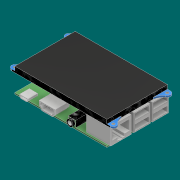
# Autodesk Inventor part: LCD
Saved by Autodesk Inventor 2018 (Build 220112000, 112)
## iProperties
Created: 2019-02-15
Part Number: LCD
Material: Generic
Document SubType Name: Modeling
Designer: Santiago
Density: 1 g/cm^3
Appearance: Default
Author: Santiago
Autodesk Inventor part; units mm, degrees
ref_plane "YZ Plane" through (0, 0, 0) normal (1, 0, 0) x (0, 1, 0)
ref_plane "XZ Plane" through (0, 0, 0) normal (0, 1, 0) x (-1, 0, 0)
sketch "Sketch1" plane through (0, 0, 0) normal (0, 0, 1) x (1, 0, 0)
  line L0 (0, 0) -> (85.5, 0)
  line L1 (85.5, 0) -> (85.5, 56)
  line L2 (85.5, 56) -> (0, 56)
  line L3 (0, 56) -> (0, 0)
  dimension "d0" = 85.5
  dimension "d1" = 56
  dimension "d2" = 85.5
  constraints: 8 end point, 1 horizontal, 1 perpendicular, 1 vertical
  measures "d0" distance of L0.start L0.end
  measures "d1" distance of L0.end L1.end
  measures "d2" distance of L1.end L2.end
extrude "Extrusion1" add sketch "Sketch1" along normal blind 3.7
sketch "Sketch2" plane through (0, 0, 0) normal (0, 0, -1) x (-1, 0, 0)
  line L0 (0, 0) -> (-85.5, 0) projected
  line L1 (-85.5, 0) -> (-85.5, 56) projected
  line L2 (0, 0) -> (-85.5, 0) projected
  line L3 (-42.75, 0) -> (-42.75, -7.3321)
  line L4 (-85.5, 0) -> (-85.5, 56) projected
  line L5 (-85.5, 28) -> (-96.093, 28)
  line L6 (-42.75, 0) -> (-88.35, 0)
  circle A0 centre (-88.35, 3.05) radius 1.25
  circle A1 centre (-88.35, 52.95) radius 1.25
  circle A2 centre (2.85, 3.05) radius 1.25
  circle A3 centre (2.85, 52.95) radius 1.25
  arc A4 (2.85, 0) -> (4.3472, 5.7072) centre (2.85, 3.05) ccw
  line L7 (0, 56) -> (0, 0) projected
  line L8 (0, 56) -> (0, 0) projected
  arc A5 (0, 13.1386) -> (4.3472, 5.7072) centre (13.2145, 15.8817) ccw
  line L9 (2.85, 0) -> (0, 0)
  line L10 (0, 0) -> (0, 13.1386)
  circle A6 centre (-88.35, 3.05) radius 1.25
  arc A7 (-89.8472, 5.7072) -> (-88.35, 0) centre (-88.35, 3.05) ccw
  arc A8 (-89.8472, 5.7072) -> (-85.5, 13.1386) centre (-98.7145, 15.8817) ccw
  line L11 (-88.35, 0) -> (-85.5, 0)
  line L12 (-85.5, 0) -> (-85.5, 13.1386)
  line L13 (-85.5, 56) -> (-85.5, 0)
  line L14 (-42.75, 56) -> (-88.35, 56)
  circle A9 centre (-88.35, 52.95) radius 1.25
  circle A10 centre (2.85, 52.95) radius 1.25
  arc A11 (4.3472, 50.2928) -> (2.85, 56) centre (2.85, 52.95) ccw
  arc A12 (4.3472, 50.2928) -> (0, 42.8614) centre (13.2145, 40.1183) ccw
  line L15 (2.85, 56) -> (0, 56)
  line L16 (0, 56) -> (0, 42.8614)
  line L17 (-88.35, 56) -> (-85.5, 56)
  circle A13 centre (-88.35, 52.95) radius 1.25
  arc A14 (-88.35, 56) -> (-89.8472, 50.2928) centre (-88.35, 52.95) ccw
  arc A15 (-85.5, 42.8614) -> (-89.8472, 50.2928) centre (-98.7145, 40.1183) ccw
  line L18 (-85.5, 42.8614) -> (-85.5, 56)
  line L19 (-88.35, 56) -> (-85.5, 56)
  line L20 (0, 0) -> (-85.5, 0)
  line L21 (-85.5, 0) -> (-85.5, 56)
  line L22 (-85.5, 56) -> (0, 56) projected
  line L23 (-85.5, 56) -> (0, 56)
  line L24 (0, 56) -> (0, 0)
  dimension "d5" = 45.6
  dimension "d7" = 2.5
  constraints: 36 end point, 21 symmetric about line, 16 centre point, 16 point on circle, 5 perpendicular, 4 coincident, 3 collinear, 3 point on line, 2 horizontal, 2 midpoint, 1 tangent, 1 vertical, 13 other
  measures "d5" distance of L3.start L6.end
  measures "d7" diameter of A0
extrude "Extrusion2" add sketch "Sketch2" along normal blind 1.5
ref_plane "Work Plane1" through (0, 0, -17.5) normal (0, 0, -1) x (-1, 0, 0)
sketch "Sketch3" plane through (0, 0, -17.5) normal (0, 0, -1) x (-1, 0, 0)
  line L0 (-88.35, 0) -> (2.85, 0) projected
  line L1 (2.85, 56) -> (-88.35, 56) projected
  line L2 (0, 13.1386) -> (0, 42.8614) projected
  line L3 (-85.5, 42.8614) -> (-85.5, 13.1386) projected
  line L4 (0, 13.1386) -> (0, 0) projected
  line L5 (-85.5, 0) -> (-85.5, 13.1386) projected
  line L6 (-85.5, 42.8614) -> (-85.5, 56) projected
  line L7 (0, 56) -> (0, 42.8614) projected
extrude "Extrusion3" add sketch "Sketch3" along normal blind 1.3
sketch "Sketch4" plane through (0, 0, -17.5) normal (0, 0, 1) x (1, 0, 0)
  line L0 (85.5, 56) -> (0, 56) projected
  line L1 (0, 56) -> (6.8, 56)
  line L2 (6.8, 56) -> (6.8, 55.5)
  line L3 (6.8, 55.5) -> (58.8, 55.5)
  line L4 (58.8, 55.5) -> (58.8, 50.5)
  line L5 (58.8, 50.5) -> (6.8, 50.5)
  line L6 (6.8, 50.5) -> (6.8, 55.5)
  point P0 (0, 0)
  dimension "d13" = 6.8
  dimension "d14" = 0.5
  dimension "d15" = 52
  dimension "d16" = 5
  dimension "d17" = 52
  constraints: 12 end point, 2 perpendicular, 1 horizontal, 1 point on line, 1 vertical
  measures "d13" distance of L0.end L1.end
  measures "d14" distance of L1.end L2.end
  measures "d15" distance of L2.end L3.end
  measures "d16" distance of L3.end L4.end
  measures "d17" distance of L4.end L5.end
extrude "Extrusion4" add sketch "Sketch4" along normal blind 16
sketch "Sketch5" plane through (85.5, 0, -17.5) normal (1, 0, 0) x (0, 0, -1)
  line L0 (0, 0) -> (0, 56) projected
  line L1 (0, 56) -> (0, 55)
  line L2 (0, 55.5) -> (0, 50.5) projected
  line L3 (0, 55) -> (0, 40)
  line L4 (0, 40) -> (-15.9, 40)
  line L5 (-15.9, 40) -> (-15.9, 55)
  line L6 (-15.9, 55) -> (0, 55)
  line L7 (-1, 41) -> (-1, 54)
  line L8 (-14.9, 54) -> (-14.9, 41)
  line L9 (-9.65, 54) -> (-9.65, 41)
  line L10 (-6.25, 54) -> (-6.25, 41)
  line L11 (-14.9, 41) -> (-9.65, 41)
  line L12 (-6.25, 41) -> (-1, 41)
  line L13 (-1, 54) -> (-6.25, 54)
  line L14 (-9.65, 54) -> (-14.9, 54)
  line L15 (0, 40) -> (0, 36.9)
  line L16 (0, 39.0096) -> (0, 38.0096)
  line L17 (0, 38.0096) -> (0, 23.0096)
  line L18 (0, 23.0096) -> (-15.9, 23.0096)
  line L19 (-15.9, 23.0096) -> (-15.9, 38.0096)
  line L20 (-15.9, 38.0096) -> (0, 38.0096)
  line L21 (-1, 24.0096) -> (-1, 37.0096)
  line L22 (-14.9, 37.0096) -> (-14.9, 24.0096)
  line L23 (-9.65, 37.0096) -> (-9.65, 24.0096)
  line L24 (-6.25, 37.0096) -> (-6.25, 24.0096)
  line L25 (-14.9, 24.0096) -> (-9.65, 24.0096)
  line L26 (-6.25, 24.0096) -> (-1, 24.0096)
  line L27 (-1, 37.0096) -> (-6.25, 37.0096)
  line L28 (-9.65, 37.0096) -> (-14.9, 37.0096)
  line L29 (0, 23.0096) -> (0, 19.9096)
  point P0 (-17.5, 0)
  dimension "d20" = 1
  dimension "d21" = 15
  dimension "d22" = 15.9
  dimension "d23" = 15
  dimension "d27" = 3.1
  dimension "d28" = 1
  dimension "d29" = 15
  dimension "d30" = 15.9
  dimension "d31" = 15
  dimension "d32" = 3.1
  constraints: 56 end point, 6 perpendicular, 3 point on line, 2 vertical
  measures "d20" distance of L0.end L1.end
  measures "d21" distance of L1.end L3.end
  measures "d22" distance of L3.end L4.end
  measures "d23" distance of L4.end L5.end
  measures "d27" distance of L3.end L15.end
  measures "d28" distance of L16.start L17.start
  measures "d29" distance of L17.start L17.end
  measures "d30" distance of L17.end L19.start
  measures "d31" distance of L19.start L19.end
  measures "d32" distance of L17.end L29.end
extrude "Extrusion5" add sketch "Sketch5" along normal blind 2
sketch "Sketch6" plane through (87.5, 0, -17.5) normal (1, 0, 0) x (0, 0, -1)
  line L0 (-9.65, 24.0096) -> (-14.9, 24.0096) projected
  line L1 (-14.9, 24.0096) -> (-14.9, 37.0096) projected
  line L2 (-14.9, 37.0096) -> (-9.65, 37.0096) projected
  line L3 (-9.65, 37.0096) -> (-9.65, 24.0096) projected
  line L4 (-1, 24.0096) -> (-6.25, 24.0096) projected
  line L5 (-6.25, 24.0096) -> (-6.25, 37.0096) projected
  line L6 (-6.25, 37.0096) -> (-1, 37.0096) projected
  line L7 (-1, 37.0096) -> (-1, 24.0096) projected
  line L8 (0, 23.0096) -> (0, 38.0096) projected
  line L9 (0, 38.0096) -> (-15.9, 38.0096) projected
  line L10 (-15.9, 38.0096) -> (-15.9, 23.0096) projected
  line L11 (-15.9, 23.0096) -> (0, 23.0096) projected
  line L12 (-1, 41) -> (-6.25, 41) projected
  line L13 (-6.25, 41) -> (-6.25, 54) projected
  line L14 (-6.25, 54) -> (-1, 54) projected
  line L15 (-1, 54) -> (-1, 41) projected
  line L16 (-14.9, 54) -> (-9.65, 54) projected
  line L17 (-9.65, 54) -> (-9.65, 41) projected
  line L18 (-9.65, 41) -> (-14.9, 41) projected
  line L19 (-14.9, 41) -> (-14.9, 54) projected
  line L20 (0, 55) -> (-15.9, 55) projected
  line L21 (-15.9, 55) -> (-15.9, 40) projected
  line L22 (-15.9, 40) -> (0, 40) projected
  line L23 (0, 40) -> (0, 55) projected
  point P0 (-17.5, 0)
extrude "Extrusion6" add sketch "Sketch6" against normal blind 19.1
sketch "Sketch7" plane through (87.5, 0, -17.5) normal (1, 0, 0) x (0, 0, -1)
  line L0 (0, 67.2) -> (0, -11.2) projected
  line L1 (0, 0) -> (0, 23.0096) projected
  line L2 (0, 0) -> (1.3, 0) projected
  line L3 (1.3, 56) -> (1.3, 0) projected
  line L4 (0, 56) -> (1.3, 56) projected
  line L5 (0, 55) -> (0, 56) projected
  line L6 (0, 40) -> (0, 55) projected
  line L7 (0, 38.0096) -> (0, 40) projected
  line L8 (0, 23.0096) -> (0, 38.0096) projected
  line L9 (0, 0) -> (0, 3)
  line L10 (0, 0) -> (0, 23.0096) projected
  line L11 (-3.8, 3) -> (-13.2, 3)
  line L12 (0, 3) -> (0, 19)
  line L13 (-3.8, 19) -> (-13.2, 19)
  line L14 (-15.9, 14.3) -> (-15.9, 3)
  line L15 (-13.2, 19) -> (-13.2, 3)
  line L16 (0, 19) -> (-1.3, 19)
  line L17 (-3.8, 19) -> (-3.8, 14.3)
  line L18 (-3.8, 14.3) -> (-1.3, 14.3)
  line L19 (-1.3, 14.3) -> (-1.3, 12.3)
  line L20 (-1.3, 12.3) -> (-0.65, 12.3)
  line L21 (0, 11) -> (-7.3396, 11)
  line L22 (-3.8, 3) -> (-3.8, 7.7)
  line L23 (-3.8, 7.7) -> (-1.3, 7.7)
  line L24 (-1.3, 7.7) -> (-1.3, 9.7)
  line L25 (-1.3, 9.7) -> (-0.65, 9.7)
  line L26 (0, 3) -> (0, 1.5)
  line L27 (0, 1.5) -> (-15.9, 1.5)
  line L28 (-16, 0) -> (-16, 5.7072) projected
  line L29 (-15.9, 1.5) -> (-15.9, 3)
  line L30 (0, 19) -> (0, 20.5)
  line L31 (0, 20.5) -> (-15.9, 20.5)
  line L32 (-15.9, 20.5) -> (-15.9, 19)
  line L33 (-15.9, 14.3) -> (-15.9, 19)
  line L34 (-16, 42.8614) -> (-16, 13.1386) projected
  line L35 (-13.2, 3) -> (-13.2, 19)
  line L36 (-13.2, 19) -> (-3.8, 19)
  line L37 (-3.8, 14.3) -> (-3.8, 19)
  line L38 (-3.8, 14.3) -> (-1.3, 14.3)
  line L39 (0, 12.3) -> (0, 9.7)
  line L40 (-1.3, 9.7) -> (-0.65, 9.7)
  line L41 (-1.3, 12.3) -> (-0.65, 12.3)
  line L42 (-1.3, 12.3) -> (-1.3, 14.3)
  line L43 (-3.8, 14.3) -> (-1.3, 14.3)
  line L44 (-1.3, 7.7) -> (-1.3, 9.7)
  line L45 (-3.8, 7.7) -> (-1.3, 7.7)
  line L46 (-3.8, 7.7) -> (-3.8, 3)
  line L47 (-13.2, 3) -> (-3.8, 3)
  line L48 (-0.65, 9.7) -> (-0.65, 12.3)
  line L49 (0, 9.7) -> (0, 12.3)
  point P0 (-17.5, 0)
  dimension "d37" = 3
  dimension "d38" = 15.9
  dimension "d39" = 16
  dimension "d40" = 15.9
  dimension "d42" = 3.8
  dimension "d43" = 4.7
  dimension "d44" = 2.5
  dimension "d45" = 2
  dimension "d46" = 1.5
  dimension "d47" = 1.5
  constraints: 76 end point, 15 perpendicular, 10 collinear, 7 point on line, 5 symmetric about line, 1 horizontal, 1 midpoint, 1 parallel
  measures "d37" distance of L1.start L9.end
  measures "d38" distance of L9.end L14.end
  measures "d39" distance of L9.end L12.end
  measures "d40" distance of L12.end L32.end
  measures "d42" distance of L13.start L12.end
  measures "d43" distance of L13.start L17.end
  measures "d44" distance of L17.end L18.end
  measures "d45" distance of L18.end L19.end
  measures "d46" distance of L9.end L26.end
  measures "d47" distance of L12.end L30.end
extrude "Extrusion7" add sketch "Sketch7" against normal blind 21.5 contours L27 L29 L14 L33 L32 L31 L0
sketch "Sketch8" plane through (66, 0, -17.5) normal (-1, 0, 0) x (0, 0, 1)
  line L0 (3.8, 19) -> (13.2, 19) projected
  line L1 (13.2, 19) -> (13.2, 3) projected
  line L2 (13.2, 3) -> (3.8, 3) projected
  line L3 (3.8, 3) -> (3.8, 7.7) projected
  line L4 (3.8, 7.7) -> (1.3, 7.7) projected
  line L5 (1.3, 7.7) -> (1.3, 9.7) projected
  line L6 (1.3, 9.7) -> (0.65, 9.7) projected
  line L7 (0.65, 9.7) -> (0.65, 12.3) projected
  line L8 (0.65, 12.3) -> (1.3, 12.3) projected
  line L9 (1.3, 12.3) -> (1.3, 14.3) projected
  line L10 (1.3, 14.3) -> (3.8, 14.3) projected
  line L11 (3.8, 14.3) -> (3.8, 19) projected
  line L12 (0, 1.5) -> (0, 20.5) projected
  line L13 (0, 1.5) -> (15.9, 1.5) projected
  line L14 (15.9, 1.5) -> (15.9, 20.5) projected
  line L15 (15.9, 20.5) -> (0, 20.5) projected
  point P0 (17.5, 0)
extrude "Extrusion8" add sketch "Sketch8" along normal blind 1 contours L0 L1 L2 L3 L4 L5 L6 L7 L8 L9 L10 L11 | L12 L15 L14 L13
sketch "Sketch9" plane through (68.4, 0, -17.5) normal (-1, 0, 0) x (0, 0, 1)
  line L0 (1, 24.0096) -> (1, 37.0096) projected
  line L1 (1, 37.0096) -> (6.25, 37.0096) projected
  line L2 (6.25, 37.0096) -> (6.25, 24.0096) projected
  line L3 (6.25, 24.0096) -> (1, 24.0096) projected
  line L4 (9.65, 24.0096) -> (9.65, 37.0096) projected
  line L5 (9.65, 37.0096) -> (14.9, 37.0096) projected
  line L6 (14.9, 37.0096) -> (14.9, 24.0096) projected
  line L7 (14.9, 24.0096) -> (9.65, 24.0096) projected
  line L8 (0, 23.0096) -> (0, 38.0096) projected
  line L9 (0, 23.0096) -> (15.9, 23.0096) projected
  line L10 (15.9, 23.0096) -> (15.9, 38.0096) projected
  line L11 (15.9, 38.0096) -> (0, 38.0096) projected
  line L12 (14.9, 54) -> (14.9, 41) projected
  line L13 (14.9, 41) -> (9.65, 41) projected
  line L14 (9.65, 41) -> (9.65, 54) projected
  line L15 (9.65, 54) -> (14.9, 54) projected
  line L16 (1, 41) -> (1, 54) projected
  line L17 (1, 54) -> (6.25, 54) projected
  line L18 (6.25, 54) -> (6.25, 41) projected
  line L19 (6.25, 41) -> (1, 41) projected
  line L20 (15.9, 55) -> (0, 55) projected
  line L21 (0, 40) -> (0, 55) projected
  line L22 (0, 40) -> (15.9, 40) projected
  line L23 (15.9, 40) -> (15.9, 55) projected
  point P0 (17.5, 0)
extrude "Extrusion9" add sketch "Sketch9" along normal blind 1 contours L0 L1 L2 L3 | L4 L5 L6 L7 | L8 L11 L10 L9 | L12 L13 L14 L15 | L16 L17 L18 L19 | L23 L22 L21 L20
sketch "Sketch10" plane through (0, 0, -17.5) normal (0, -1, 0) x (1, 0, 0)
  line L0 (65, 0) -> (65, 15.9) projected
  line L1 (65, 0) -> (56.5, 0)
  line L2 (0, 0) -> (85.5, 0) projected
  line L3 (56.5, 0) -> (56.5, 6)
  line L4 (56.5, 6) -> (49.5, 6)
  line L5 (49.5, 6) -> (49.5, 0)
  line L6 (56.5, 0) -> (49.5, 0)
  line L7 (58.8, 0) -> (6.8, 0) projected
  point P0 (0, 17.5)
  dimension "d54" = 8.5
  dimension "d55" = 6
  dimension "d56" = 7
  constraints: 10 end point, 3 perpendicular, 2 point on line, 1 collinear
  measures "d54" distance of L0.start L1.end
  measures "d55" distance of L1.end L3.end
  measures "d56" distance of L3.end L4.end
extrude "Extrusion10" add sketch "Sketch10" against normal blind 18
sketch "Sketch11" plane through (0, 0, -18.8) normal (0, -1, 0) x (1, 0, 0)
  circle A0 centre (53, 4.3) radius 3
  circle A1 centre (53, 4.3) radius 1.7979
  point P0 (0, 18.8)
  dimension "d59" = 6
  constraints: 2 centre point
  measures "d59" diameter of A0
extrude "Extrusion11" add sketch "Sketch11" along normal blind 2
sketch "Sketch12" plane through (0, 0, -18.8) normal (0, -1, 0) x (1, 0, 0)
  line L0 (49.5, 7.3) -> (49.5, 1.3) projected
  line L1 (49.5, 7.3) -> (49.5, 8.3)
  line L2 (49.5, 8.3) -> (39.5, 8.3)
  line L3 (39.5, 8.3) -> (39.5, 4.3)
  arc A0 (39.5, 4.3) -> (36.9589, 1.3) centre (42.1902, -0.5548) ccw
  line L4 (39.5, 8.3) -> (24.5, 8.3)
  line L5 (24.5, 8.3) -> (24.5, 4.3)
  line L6 (32, 8.3) -> (32, 11.2612)
  arc A1 (27.0411, 1.3) -> (24.5, 4.3) centre (21.8098, -0.5548) ccw
  line L7 (27.0411, 1.3) -> (36.9589, 1.3)
  line L8 (0, 1.3) -> (49.5, 1.3) projected
  line L9 (25.5, 7.3) -> (38.5, 7.3)
  line L10 (38.5, 7.3) -> (38.5, 4.8572)
  arc A2 (38.5, 4.8572) -> (36.2947, 2.3) centre (42.1902, -0.5548) ccw
  line L11 (36.2947, 2.3) -> (27.7053, 2.3)
  arc A3 (27.7053, 2.3) -> (25.5, 4.8572) centre (21.8098, -0.5548) ccw
  line L12 (25.5, 4.8572) -> (25.5, 7.3)
  point P0 (0, 18.8)
  dimension "d62" = 1
  dimension "d63" = 10
  dimension "d64" = 4
  dimension "d65" = 15
  dimension "d66" = 1
  constraints: 22 end point, 8 point on circle, 4 centre point, 4 perpendicular, 2 symmetric about line, 2 vertical, 1 collinear, 1 horizontal, 1 midpoint, 6 other
  measures "d62" distance of L0.start L1.end
  measures "d63" distance of L1.end L2.end
  measures "d64" distance of L2.end L3.end
  measures "d65" distance of L2.end L4.end
  measures "d66" distance between parallel lines of L4 L9
extrude "Extrusion12" add sketch "Sketch12" against normal blind 10 contours L7 A1 L5 L4 L3 A0
sketch "Sketch13" plane through (0, 0, -18.8) normal (0, -1, 0) x (1, 0, 0)
  arc A0 (27.0411, 1.3) -> (24.5, 4.3) centre (21.8098, -0.5548) ccw projected
  line L0 (24.5, 4.3) -> (24.5, 8.3) projected
  line L1 (24.5, 8.3) -> (39.5, 8.3) projected
  line L2 (36.2947, 2.3) -> (27.7053, 2.3) projected
  arc A1 (27.7053, 2.3) -> (25.5, 4.8572) centre (21.8098, -0.5548) ccw projected
  line L3 (25.5, 4.8572) -> (25.5, 7.3) projected
  line L4 (25.5, 7.3) -> (38.5, 7.3) projected
  line L5 (38.5, 7.3) -> (38.5, 4.8572) projected
  arc A2 (38.5, 4.8572) -> (36.2947, 2.3) centre (42.1902, -0.5548) ccw projected
  arc A3 (39.5, 4.3) -> (36.9589, 1.3) centre (42.1902, -0.5548) ccw projected
  line L6 (39.5, 8.3) -> (39.5, 4.3) projected
  arc A4 (27.0411, 1.3) -> (24.5, 4.3) centre (21.8098, -0.5548) ccw projected
  line L7 (36.9589, 1.3) -> (49.5, 1.3) projected
  line L8 (27.0411, 1.3) -> (36.9589, 1.3)
  point P0 (0, 18.8)
  constraints: 2 end point, 1 horizontal
extrude "Extrusion13" add sketch "Sketch13" along normal blind 2
sketch "Sketch14" plane through (0, 10, -18.8) normal (0, 1, 0) x (1, 0, 0)
  line L0 (25.5, -7.3) -> (25.5, -4.8572) projected
  arc A0 (25.5, -4.8572) -> (27.7053, -2.3) centre (21.8098, 0.5548) ccw projected
  line L1 (27.7053, -2.3) -> (36.2947, -2.3) projected
  arc A1 (36.2947, -2.3) -> (38.5, -4.8572) centre (42.1902, 0.5548) ccw projected
  line L2 (38.5, -4.8572) -> (38.5, -7.3) projected
  line L3 (38.5, -7.3) -> (25.5, -7.3) projected
  line L4 (39.5, -8.3) -> (39.5, -4.3) projected
  arc A2 (36.9589, -1.3) -> (39.5, -4.3) centre (42.1902, 0.5548) ccw projected
  line L5 (27.0411, -1.3) -> (36.9589, -1.3) projected
  arc A3 (24.5, -4.3) -> (27.0411, -1.3) centre (21.8098, 0.5548) ccw projected
  line L6 (24.5, -4.3) -> (24.5, -8.3) projected
  line L7 (24.5, -8.3) -> (39.5, -8.3) projected
  point P0 (0, -18.8)
extrude "Extrusion14" add sketch "Sketch14" along normal blind 1 contours L0 A0 L1 A1 L2 L3 | L7 L6 A3 L5 A2 L4
sketch "Sketch15" plane through (0, 10, -18.8) normal (0, -1, 0) x (1, 0, 0)
  line L0 (25.5, 4.8572) -> (25.5, 7.3) projected
  line L1 (38.5, 7.3) -> (38.5, 4.8572) projected
  line L2 (38.5, 4.8572) -> (25.5, 4.8572)
  line L3 (27.7053, 4.8572) -> (27.7053, 5.8572)
  line L4 (27.7053, 5.8572) -> (36.2947, 5.8572)
  line L5 (36.2947, 5.8572) -> (36.2947, 4.8572)
  point P0 (0, 18.8)
  dimension "d73" = 1
  constraints: 8 end point, 2 point on line, 1 horizontal, 1 parallel, 1 perpendicular, 1 vertical
  measures "d73" distance of L3.start L3.end
extrude "Extrusion15" add sketch "Sketch15" along normal blind 10
sketch "Sketch16" plane through (53, 0, -14.5) normal (0, -1, 0) x (1, 0, 0)
  circle A0 centre (0, 0) radius 1.7979 projected
  point P0 (-53, 14.5)
extrude "Extrusion16" cut sketch "Sketch16" against normal blind 10
sketch "Sketch17" plane through (0, -2, -18.8) normal (0, -1, 0) x (1, 0, 0)
  line L0 (24.5, 8.3) -> (24.5, 4.3) projected
  line L1 (24.5, 4.3) -> (14.3, 4.3)
  line L2 (14.3, 4.3) -> (6.5, 4.3)
  line L3 (6.5, 4.3) -> (6.5, 2.8)
  line L4 (14.3, 2.8) -> (14.3, 4.3)
  line L5 (0, 1.3) -> (27.0411, 1.3) projected
  arc A0 (12.9132, 1.3) -> (14.3, 2.8) centre (12.5923, 2.9877) ccw
  line L6 (10.4, 4.3) -> (10.4, 5.6395)
  arc A1 (6.5, 2.8) -> (7.8868, 1.3) centre (8.2077, 2.9877) ccw
  line L7 (12.9132, 1.3) -> (7.8868, 1.3)
  line L8 (7.1, 3.7) -> (13.7, 3.7)
  line L9 (13.7, 3.7) -> (13.7, 2.8364)
  arc A2 (12.8505, 1.9) -> (13.7, 2.8364) centre (12.5923, 2.9877) ccw
  line L10 (12.8505, 1.9) -> (7.9495, 1.9)
  arc A3 (7.1, 2.8364) -> (7.9495, 1.9) centre (8.2077, 2.9877) ccw
  line L11 (7.1, 2.8364) -> (7.1, 3.7)
  point P0 (0, 18.8)
  dimension "d78" = 10.2
  dimension "d79" = 7.8
  dimension "d80" = 1.5
  dimension "d81" = 0.6
  constraints: 20 end point, 8 point on circle, 4 centre point, 2 perpendicular, 2 point on line, 2 symmetric about line, 1 collinear, 1 horizontal, 1 midpoint, 1 vertical, 6 other
  measures "d78" distance of L0.end L1.end
  measures "d79" distance of L1.end L2.end
  measures "d80" distance of L2.end L3.end
  measures "d81" distance between parallel lines of L2 L8
extrude "Extrusion17" add sketch "Sketch17" against normal blind 8
sketch "Sketch18" plane through (0, 6, -18.8) normal (0, 1, 0) x (1, 0, 0)
  line L0 (7.1, -3.7) -> (7.1, -2.8364) projected
  arc A0 (7.9495, -1.9) -> (7.1, -2.8364) centre (8.2077, -2.9877) ccw projected
  line L1 (7.9495, -1.9) -> (12.8505, -1.9) projected
  arc A1 (13.7, -2.8364) -> (12.8505, -1.9) centre (12.5923, -2.9877) ccw projected
  line L2 (13.7, -2.8364) -> (13.7, -3.7) projected
  line L3 (13.7, -3.7) -> (7.1, -3.7) projected
  line L4 (6.5, -4.3) -> (14.3, -4.3) projected
  line L5 (14.3, -4.3) -> (14.3, -2.8) projected
  arc A2 (14.3, -2.8) -> (12.9132, -1.3) centre (12.5923, -2.9877) ccw projected
  line L6 (7.8868, -1.3) -> (12.9132, -1.3) projected
  arc A3 (7.8868, -1.3) -> (6.5, -2.8) centre (8.2077, -2.9877) ccw projected
  line L7 (6.5, -2.8) -> (6.5, -4.3) projected
  point P0 (0, -18.8)
extrude "Extrusion18" add sketch "Sketch18" along normal blind 1 contours L0 A0 L1 A1 L2 L3 | L7 A3 L6 A2 L5 L4
sketch "Sketch19" plane through (0, 0, -17.5) normal (0, 0, 1) x (1, 0, 0)
  line L0 (0, 56) -> (0, 0) projected
  line L1 (0, 28) -> (2, 28)
  line L2 (2, 28) -> (2, 18)
  line L3 (2, 18) -> (5, 18)
  line L4 (5, 18) -> (5, 38)
  line L5 (5, 38) -> (2, 38)
  line L6 (2, 38) -> (2, 28)
  dimension "d86" = 2
  dimension "d87" = 10
  dimension "d88" = 3
  dimension "d89" = 20
  constraints: 12 end point, 4 perpendicular, 1 collinear, 1 horizontal, 1 midpoint, 1 point on line
  measures "d86" distance of L1.start L1.end
  measures "d87" distance of L1.end L2.end
  measures "d88" distance of L2.end L3.end
  measures "d89" distance of L3.end L4.end
extrude "Extrusion19" add sketch "Sketch19" along normal blind 5
sketch "Sketch20" plane through (0, 0, -17.5) normal (0, 0, 1) x (1, 0, 0)
  line L0 (12.5918, 44.0351) -> (31.8728, 44.0351)
  line L1 (31.8728, 44.0351) -> (31.8728, 30.1324)
  line L2 (12.5918, 44.0351) -> (12.5918, 30.1324)
  line L3 (12.5918, 30.1324) -> (31.8728, 30.1324)
  point P0 (0, 0)
  constraints: 8 end point, 2 perpendicular, 1 horizontal, 1 vertical
extrude "Extrusion20" add sketch "Sketch20" along normal blind 1
sketch "Sketch21" plane through (68.4, 0, -17.5) normal (1, 0, 0) x (0, 0, -1)
  line L0 (-14.9, 24.0096) -> (-9.65, 24.0096) projected
  line L1 (-9.65, 24.0096) -> (-9.65, 37.0096) projected
  line L2 (-9.65, 37.0096) -> (-14.9, 37.0096) projected
  line L3 (-14.9, 37.0096) -> (-14.9, 24.0096) projected
  line L4 (-9.65, 54) -> (-14.9, 54) projected
  line L5 (-14.9, 54) -> (-14.9, 41) projected
  line L6 (-14.9, 41) -> (-9.65, 41) projected
  line L7 (-9.65, 41) -> (-9.65, 54) projected
  line L8 (-6.25, 41) -> (-1, 41) projected
  line L9 (-1, 41) -> (-1, 54) projected
  line L10 (-1, 54) -> (-6.25, 54) projected
  line L11 (-6.25, 54) -> (-6.25, 41) projected
  line L12 (-6.25, 24.0096) -> (-1, 24.0096) projected
  line L13 (-1, 24.0096) -> (-1, 37.0096) projected
  line L14 (-1, 37.0096) -> (-6.25, 37.0096) projected
  line L15 (-6.25, 37.0096) -> (-6.25, 24.0096) projected
  line L16 (-9.65, 24.0096) -> (-14.9, 24.0096) projected
  line L17 (-12.275, 24.0096) -> (-12.275, 37.0096)
  line L18 (-12.275, 37.0096) -> (-13.475, 37.0096)
  line L19 (-9.65, 37.0096) -> (-14.9, 37.0096) projected
  line L20 (-13.475, 37.0096) -> (-13.475, 24.0096)
  line L21 (-12.275, 24.0096) -> (-13.475, 24.0096)
  line L22 (-12.275, 41) -> (-12.275, 54)
  line L23 (-13.475, 54) -> (-13.475, 41)
  line L24 (-3.625, 24.0096) -> (-3.625, 37.0096)
  line L25 (-4.825, 37.0096) -> (-4.825, 24.0096)
  line L26 (-3.625, 41) -> (-3.625, 54)
  line L27 (-4.825, 54) -> (-4.825, 41)
  line L28 (-4.825, 24.0096) -> (-3.625, 24.0096)
  line L29 (-6.25, 24.0096) -> (-1, 24.0096) projected
  line L30 (-4.825, 37.0096) -> (-3.625, 37.0096)
  line L31 (-13.475, 41) -> (-12.275, 41)
  line L32 (-13.475, 54) -> (-12.275, 54)
  line L33 (-9.65, 54) -> (-14.9, 54) projected
  line L34 (-4.825, 54) -> (-3.625, 54)
  line L35 (-4.825, 41) -> (-3.625, 41)
  point P0 (-17.5, 0)
  dimension "d94" = 1.2
  dimension "d95" = 1.2
  dimension "d96" = 1.2
  dimension "d97" = 1.2
  constraints: 32 end point, 6 collinear, 2 midpoint, 2 point on line, 1 parallel, 1 perpendicular
  measures "d94" distance of L17.end L18.end
  measures "d95" distance of L22.end L23.start
  measures "d96" distance of L24.end L25.start
  measures "d97" distance of L26.end L27.start
extrude "Extrusion21" add sketch "Sketch21" along normal blind 15 contours L20 L2 L17 L0 | L22 L6 L23 L4 | L27 L10 L26 L8 | L25 L14 L24 L12
body "Solid1"
